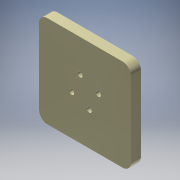
# Autodesk Inventor part: 실리콘틀_밑판
Saved by Autodesk Inventor 2017 (Build 210142000, 142)
## iProperties
Part Number: 실리콘틀_밑판
Material: 나일론, 이황화 몰리브덴
Document SubType Name: Modeling
Designer: minom
Mass: 136.73 g
Surface Area: 286 cm^2
Volume: 121 cm^3
Density: 1.13 g/cm^3
Appearance: 나일론 6
Author: minom
Autodesk Inventor part; units mm, degrees
ref_plane "YZ Plane" through (0, 0, 0) normal (1, 0, 0) x (0, 1, 0)
ref_plane "XZ Plane" through (0, 0, 0) normal (0, 1, 0) x (-1, 0, 0)
ref_plane "XY Plane" through (0, 0, 0) normal (0, 0, 1) x (1, 0, 0)
sketch "스케치1" plane through (0, 0, 0) normal (0, 1, 0) x (-1, 0, 0)
  line L0 (55, 55) -> (-55, 55)
  line L1 (-55, 55) -> (-55, -55)
  line L2 (-55, -55) -> (55, -55)
  line L3 (55, -55) -> (55, 55)
  point P0 (0, 0)
  dimension "d0" = 110
  dimension "d1" = 110
  dimension "d2" = 55
  dimension "d3" = 55
  constraints: 8 end point, 2 parallel, 1 horizontal, 1 perpendicular
  measures "d0" distance of L2.end L1.end
  measures "d1" distance of L1.end L0.end
  measures "d2" distance from line of L1 point (0, 0)
  measures "d3" distance from line of L2 point (0, 0)
extrude "돌출1" add sketch "스케치1" against normal blind 10
sketch "스케치2" plane through (0, 0, 0) normal (0, 1, 0) x (1, 0, 0)
  circle A0 centre (0, 0) radius 33.5 projected
  circle A1 centre (0, 0) radius 38.5 projected
  circle A2 centre (0, 0) radius 43.5 projected
  line L0 (-55, -55) -> (55, -55) projected
  line L1 (55, -55) -> (55, 55) projected
  line L2 (55, 55) -> (-55, 55) projected
  line L3 (-55, 55) -> (-55, -55) projected
extrude "돌출2" add sketch "스케치2" along normal blind 2
sketch "스케치3" plane through (0, 0, 0) normal (0, 1, 0) x (1, 0, 0)
  circle A0 centre (0, 0) radius 33.5 projected
  circle A1 centre (-16, 7) radius 3
  circle A2 centre (5, 15) radius 3
  circle A3 centre (16, -7) radius 3
  circle A4 centre (-6, -16) radius 3
  dimension "d8" = 6
  dimension "d9" = 6
  dimension "d10" = 6
  dimension "d11" = 6
  constraints: 4 centre point
  measures "d8" diameter of A1
  measures "d9" diameter of A2
  measures "d10" diameter of A3
  measures "d11" diameter of A4
extrude "돌출3" cut sketch "스케치3" against normal blind 10 contours A1 | A2 | A3 | A4
fillet "모깎기1" radius 10 4 edges at (-55, -4, -55) (55, -4, -55) (55, -4, 55) (-55, -4, 55)
sketch "스케치5" plane through (0, 2, 0) normal (0, 1, 0) x (1, 0, 0)
  circle A0 centre (0, 0) radius 43.5 projected
  arc A1 (-55, -45) -> (-45, -55) centre (-45, -45) ccw projected
  line L0 (-45, -55) -> (45, -55) projected
  arc A2 (45, -55) -> (55, -45) centre (45, -45) ccw projected
  line L1 (55, -45) -> (55, 45) projected
  arc A3 (55, 45) -> (45, 55) centre (45, 45) ccw projected
  line L2 (45, 55) -> (-45, 55) projected
  arc A4 (-45, 55) -> (-55, 45) centre (-45, 45) ccw projected
  line L3 (-55, 45) -> (-55, -45) projected
  circle A5 centre (0, 0) radius 38.5 projected
  circle A6 centre (0, 0) radius 43.5 projected
  circle A7 centre (0, 0) radius 45.5
  dimension "d18" = 91
  constraints: 1 centre point, 1 coincident
  measures "d18" diameter of A7
extrude "돌출5" cut sketch "스케치5" against normal blind 2 contours A7
